Autodesk Fusion 360 part; units mm, degrees
(part 3 of 3)
  spline S31 degree 5 poles (22.8468, -21.88) (22.8333, -21.884) (22.8062, -21.8919) (22.7658, -21.904) (22.7119, -21.9202) (22.6448, -21.9407) (22.5778, -21.9615) (22.5111, -21.9825) (22.4444, -22.0039) (22.378, -22.0255) (22.3118, -22.0473) (22.2457, -22.0695) (22.1798, -22.0919) (22.1141, -22.1146) (22.0486, -22.1375) (21.9832, -22.1608) (21.9181, -22.1843) (21.8531, -22.2081) (21.7884, -22.2321) (21.7238, -22.2565) (21.6595, -22.2811) (21.5953, -22.306) (21.5314, -22.3312) (21.4676, -22.3567) (21.4041, -22.3825) (21.3408, -22.4086) (21.2777, -22.4349) (21.2148, -22.4616) (21.1522, -22.4885) (21.0897, -22.5157) (21.0275, -22.5433) (20.9655, -22.5711) (20.9038, -22.5992) (20.8423, -22.6276) (20.781, -22.6564) (20.72, -22.6854) (20.6592, -22.7148) (20.5987, -22.7444) (20.5384, -22.7744) (20.4784, -22.8047) (20.4187, -22.8353) (20.3592, -22.8662) (20.3, -22.8975) (20.2411, -22.9291) (20.1825, -22.9611) (20.1241, -22.9933) (20.066, -23.0259) (20.0083, -23.0589) (19.9508, -23.0921) (19.8936, -23.1258) (19.8368, -23.1598) (19.7803, -23.1942) (19.7242, -23.2289) (19.6685, -23.2641) (19.6131, -23.2997) (19.558, -23.3357) (19.5033, -23.372) (19.4489, -23.4086) (19.3948, -23.4456) (19.3412, -23.4831) (19.288, -23.521) (19.2355, -23.5596) (19.1835, -23.5987) (19.1321, -23.6385) (19.0813, -23.6788) (19.0309, -23.7195) (18.9808, -23.7605) (18.931, -23.8018) (18.8816, -23.8435) (18.8331, -23.886) (18.7858, -23.9297) (18.7495, -23.9661) (18.7233, -23.9943) (18.7062, -24.0136) (18.6978, -24.0233) knots -1 -1 -1 -1 -1 -1 -0.98571429 -0.97142857 -0.95714286 -0.94285714 -0.92857143 -0.91428571 -0.9 -0.88571429 -0.87142857 -0.85714286 -0.84285714 -0.82857143 -0.81428571 -0.8 -0.78571429 -0.77142857 -0.75714286 -0.74285714 -0.72857143 -0.71428571 -0.7 -0.68571429 -0.67142857 -0.65714286 -0.64285714 -0.62857143 -0.61428571 -0.6 -0.58571429 -0.57142857 -0.55714286 -0.54285714 -0.52857143 -0.51428571 -0.5 -0.48571429 -0.47142857 -0.45714286 -0.44285714 -0.42857143 -0.41428571 -0.4 -0.38571429 -0.37142857 -0.35714286 -0.34285714 -0.32857143 -0.31428571 -0.3 -0.28571429 -0.27142857 -0.25714286 -0.24285714 -0.22857143 -0.21428571 -0.2 -0.18571429 -0.17142857 -0.15714286 -0.14285714 -0.12857143 -0.11428571 -0.1 -0.08571429 -0.07142857 -0.05714286 -0.04285714 -0.02857143 -0.01428571 0 0 0 0 0 0
  line L31 (18.6978, -24.0233) -> (18.685, -24.0381)
  arc A63 (16.9379, -24.2063) -> (18.685, -24.0381) centre (17.7235, -23.2085) ccw
  arc A64 (16.9379, -24.2063) -> (16.3968, -23.7911) centre (0, -45.72) ccw
  arc A65 (16.1071, -22.0599) -> (16.3968, -23.7911) centre (17.1573, -22.774) ccw
  line L32 (16.1071, -22.0599) -> (16.1181, -22.0438)
  spline S32 degree 5 poles (16.1181, -22.0438) (16.1253, -22.0332) (16.1395, -22.0117) (16.16, -21.979) (16.1857, -21.9345) (16.2157, -21.8776) (16.2441, -21.8197) (16.2717, -21.7613) (16.2986, -21.7025) (16.3253, -21.6434) (16.3515, -21.5842) (16.3773, -21.5247) (16.4024, -21.4648) (16.4268, -21.4044) (16.4504, -21.3437) (16.4733, -21.2825) (16.4956, -21.221) (16.5174, -21.1592) (16.5387, -21.0972) (16.5596, -21.0349) (16.5801, -20.9724) (16.6001, -20.9097) (16.6197, -20.8468) (16.6388, -20.7836) (16.6574, -20.7201) (16.6755, -20.6564) (16.6932, -20.5925) (16.7105, -20.5284) (16.7273, -20.464) (16.7438, -20.3995) (16.7599, -20.3348) (16.7755, -20.2699) (16.7908, -20.2048) (16.8057, -20.1395) (16.8202, -20.0741) (16.8343, -20.0085) (16.848, -19.9426) (16.8614, -19.8767) (16.8743, -19.8105) (16.887, -19.7442) (16.8992, -19.6778) (16.9111, -19.6112) (16.9227, -19.5444) (16.9339, -19.4775) (16.9447, -19.4104) (16.9552, -19.3432) (16.9653, -19.2758) (16.9751, -19.2083) (16.9846, -19.1407) (16.9937, -19.0729) (17.0025, -19.005) (17.011, -18.937) (17.0191, -18.8688) (17.0269, -18.8005) (17.0343, -18.7321) (17.0415, -18.6636) (17.0483, -18.5949) (17.0548, -18.5262) (17.0609, -18.4573) (17.0668, -18.3883) (17.0723, -18.3191) (17.0776, -18.2499) (17.0825, -18.1806) (17.0871, -18.1111) (17.0913, -18.0416) (17.0953, -17.9719) (17.099, -17.9021) (17.1023, -17.8323) (17.1054, -17.7623) (17.1081, -17.6923) (17.1106, -17.6221) (17.1123, -17.5659) (17.1134, -17.5237) (17.1142, -17.4956) (17.1145, -17.4815) knots 0 0 0 0 0 0 0.01428571 0.02857143 0.04285714 0.05714286 0.07142857 0.08571429 0.1 0.11428571 0.12857143 0.14285714 0.15714286 0.17142857 0.18571429 0.2 0.21428571 0.22857143 0.24285714 0.25714286 0.27142857 0.28571429 0.3 0.31428571 0.32857143 0.34285714 0.35714286 0.37142857 0.38571429 0.4 0.41428571 0.42857143 0.44285714 0.45714286 0.47142857 0.48571429 0.5 0.51428571 0.52857143 0.54285714 0.55714286 0.57142857 0.58571429 0.6 0.61428571 0.62857143 0.64285714 0.65714286 0.67142857 0.68571429 0.7 0.71428571 0.72857143 0.74285714 0.75714286 0.77142857 0.78571429 0.8 0.81428571 0.82857143 0.84285714 0.85714286 0.87142857 0.88571429 0.9 0.91428571 0.92857143 0.94285714 0.95714286 0.97142857 0.98571429 1 1 1 1 1 1
  arc A66 (17.1145, -17.4815) -> (15.898, -16.7791) centre (0, -45.72) ccw
  spline S33 degree 5 poles (15.898, -16.7791) (15.886, -16.7865) (15.862, -16.8012) (15.826, -16.8233) (15.7782, -16.8528) (15.7187, -16.89) (15.6594, -16.9275) (15.6003, -16.9651) (15.5415, -17.0029) (15.4829, -17.041) (15.4246, -17.0792) (15.3665, -17.1177) (15.3086, -17.1564) (15.251, -17.1954) (15.1937, -17.2345) (15.1366, -17.2739) (15.0797, -17.3134) (15.0232, -17.3532) (14.9669, -17.3932) (14.9108, -17.4335) (14.855, -17.4739) (14.7995, -17.5146) (14.7443, -17.5555) (14.6893, -17.5966) (14.6346, -17.6379) (14.5802, -17.6795) (14.5261, -17.7213) (14.4722, -17.7633) (14.4187, -17.8055) (14.3654, -17.848) (14.3124, -17.8907) (14.2598, -17.9336) (14.2074, -17.9767) (14.1554, -18.0201) (14.1036, -18.0637) (14.0522, -18.1076) (14.0011, -18.1517) (13.9503, -18.196) (13.8998, -18.2405) (13.8497, -18.2853) (13.7999, -18.3303) (13.7505, -18.3756) (13.7014, -18.4211) (13.6527, -18.4669) (13.6043, -18.5129) (13.5563, -18.5592) (13.5087, -18.6057) (13.4614, -18.6525) (13.4145, -18.6995) (13.368, -18.7468) (13.3219, -18.7943) (13.2762, -18.8422) (13.231, -18.8903) (13.1863, -18.9387) (13.142, -18.9874) (13.0981, -19.0364) (13.0546, -19.0856) (13.0116, -19.1351) (12.969, -19.1849) (12.9268, -19.2349) (12.8853, -19.2853) (12.8445, -19.3362) (12.8044, -19.3874) (12.7651, -19.4392) (12.7264, -19.4912) (12.6883, -19.5436) (12.6505, -19.5962) (12.6131, -19.649) (12.5762, -19.702) (12.5403, -19.7556) (12.506, -19.8101) (12.4803, -19.8546) (12.4622, -19.8886) (12.4508, -19.9117) (12.4452, -19.9233) knots -1 -1 -1 -1 -1 -1 -0.98571429 -0.97142857 -0.95714286 -0.94285714 -0.92857143 -0.91428571 -0.9 -0.88571429 -0.87142857 -0.85714286 -0.84285714 -0.82857143 -0.81428571 -0.8 -0.78571429 -0.77142857 -0.75714286 -0.74285714 -0.72857143 -0.71428571 -0.7 -0.68571429 -0.67142857 -0.65714286 -0.64285714 -0.62857143 -0.61428571 -0.6 -0.58571429 -0.57142857 -0.55714286 -0.54285714 -0.52857143 -0.51428571 -0.5 -0.48571429 -0.47142857 -0.45714286 -0.44285714 -0.42857143 -0.41428571 -0.4 -0.38571429 -0.37142857 -0.35714286 -0.34285714 -0.32857143 -0.31428571 -0.3 -0.28571429 -0.27142857 -0.25714286 -0.24285714 -0.22857143 -0.21428571 -0.2 -0.18571429 -0.17142857 -0.15714286 -0.14285714 -0.12857143 -0.11428571 -0.1 -0.08571429 -0.07142857 -0.05714286 -0.04285714 -0.02857143 -0.01428571 0 0 0 0 0 0
  line L33 (12.4452, -19.9233) -> (12.4367, -19.9408)
  arc A67 (10.7926, -20.5555) -> (12.4367, -19.9408) centre (11.2931, -19.3883) ccw
  arc A68 (10.7926, -20.5555) -> (10.1625, -20.2945) centre (0, -45.72) ccw
  arc A69 (9.4346, -18.6973) -> (10.1625, -20.2945) centre (10.6338, -19.1152) ccw
  line L34 (9.4346, -18.6973) -> (9.441, -18.6789)
  spline S34 degree 5 poles (9.441, -18.6789) (9.4452, -18.6667) (9.4534, -18.6423) (9.4647, -18.6055) (9.478, -18.5558) (9.4923, -18.4931) (9.5048, -18.4298) (9.5162, -18.3662) (9.5271, -18.3024) (9.5375, -18.2385) (9.5476, -18.1745) (9.5571, -18.1103) (9.5658, -18.046) (9.5738, -17.9814) (9.5808, -17.9166) (9.5871, -17.8516) (9.5927, -17.7864) (9.5978, -17.7211) (9.6023, -17.6556) (9.6064, -17.5901) (9.61, -17.5244) (9.6131, -17.4587) (9.6157, -17.3928) (9.6178, -17.3268) (9.6193, -17.2607) (9.6204, -17.1945) (9.6209, -17.1282) (9.621, -17.0618) (9.6206, -16.9953) (9.6198, -16.9287) (9.6186, -16.862) (9.6169, -16.7953) (9.6149, -16.7284) (9.6123, -16.6615) (9.6094, -16.5946) (9.606, -16.5275) (9.6023, -16.4604) (9.5981, -16.3932) (9.5935, -16.326) (9.5885, -16.2587) (9.5832, -16.1913) (9.5774, -16.1239) (9.5713, -16.0564) (9.5648, -15.9889) (9.5579, -15.9213) (9.5506, -15.8536) (9.543, -15.7859) (9.535, -15.7182) (9.5266, -15.6504) (9.5179, -15.5826) (9.5088, -15.5147) (9.4994, -15.4468) (9.4896, -15.3789) (9.4794, -15.3109) (9.4689, -15.2429) (9.4581, -15.1749) (9.4469, -15.1068) (9.4354, -15.0387) (9.4235, -14.9705) (9.4113, -14.9024) (9.3987, -14.8342) (9.3859, -14.7659) (9.3727, -14.6977) (9.3591, -14.6294) (9.3453, -14.5611) (9.3311, -14.4928) (9.3166, -14.4245) (9.3017, -14.3561) (9.2866, -14.2878) (9.2711, -14.2194) (9.2553, -14.151) (9.2424, -14.0962) (9.2326, -14.0552) (9.226, -14.0278) (9.2227, -14.0141) knots 0 0 0 0 0 0 0.01428571 0.02857143 0.04285714 0.05714286 0.07142857 0.08571429 0.1 0.11428571 0.12857143 0.14285714 0.15714286 0.17142857 0.18571429 0.2 0.21428571 0.22857143 0.24285714 0.25714286 0.27142857 0.28571429 0.3 0.31428571 0.32857143 0.34285714 0.35714286 0.37142857 0.38571429 0.4 0.41428571 0.42857143 0.44285714 0.45714286 0.47142857 0.48571429 0.5 0.51428571 0.52857143 0.54285714 0.55714286 0.57142857 0.58571429 0.6 0.61428571 0.62857143 0.64285714 0.65714286 0.67142857 0.68571429 0.7 0.71428571 0.72857143 0.74285714 0.75714286 0.77142857 0.78571429 0.8 0.81428571 0.82857143 0.84285714 0.85714286 0.87142857 0.88571429 0.9 0.91428571 0.92857143 0.94285714 0.95714286 0.97142857 0.98571429 1 1 1 1 1 1
  arc A70 (9.2227, -14.0141) -> (7.8659, -13.6506) centre (0, -45.72) ccw
  spline S35 degree 5 poles (7.8659, -13.6506) (7.8562, -13.6608) (7.8368, -13.6812) (7.8077, -13.7118) (7.7692, -13.7528) (7.7213, -13.8041) (7.6737, -13.8556) (7.6264, -13.9072) (7.5794, -13.959) (7.5327, -14.0109) (7.4862, -14.063) (7.4401, -14.1152) (7.3942, -14.1676) (7.3486, -14.2201) (7.3034, -14.2727) (7.2584, -14.3255) (7.2138, -14.3784) (7.1694, -14.4315) (7.1254, -14.4847) (7.0816, -14.5381) (7.0382, -14.5916) (6.9951, -14.6453) (6.9523, -14.6991) (6.9099, -14.753) (6.8678, -14.8071) (6.826, -14.8613) (6.7845, -14.9157) (6.7433, -14.9702) (6.7026, -15.0248) (6.6621, -15.0796) (6.622, -15.1346) (6.5822, -15.1897) (6.5428, -15.2449) (6.5038, -15.3003) (6.4651, -15.3558) (6.4268, -15.4115) (6.3888, -15.4673) (6.3512, -15.5232) (6.314, -15.5793) (6.2772, -15.6356) (6.2407, -15.6919) (6.2047, -15.7485) (6.1691, -15.8051) (6.1338, -15.862) (6.099, -15.9189) (6.0646, -15.9761) (6.0307, -16.0333) (5.9971, -16.0907) (5.964, -16.1483) (5.9313, -16.206) (5.8991, -16.2639) (5.8673, -16.3219) (5.8361, -16.3801) (5.8054, -16.4384) (5.7753, -16.4969) (5.7456, -16.5556) (5.7163, -16.6144) (5.6875, -16.6733) (5.6592, -16.7324) (5.6315, -16.7917) (5.6045, -16.8511) (5.5782, -16.9108) (5.5528, -16.9707) (5.5282, -17.0308) (5.5043, -17.0911) (5.481, -17.1516) (5.4581, -17.2122) (5.4356, -17.2728) (5.4137, -17.3336) (5.3929, -17.3947) (5.3739, -17.4561) (5.3606, -17.5058) (5.352, -17.5434) (5.3468, -17.5686) (5.3444, -17.5812) knots -1 -1 -1 -1 -1 -1 -0.98571429 -0.97142857 -0.95714286 -0.94285714 -0.92857143 -0.91428571 -0.9 -0.88571429 -0.87142857 -0.85714286 -0.84285714 -0.82857143 -0.81428571 -0.8 -0.78571429 -0.77142857 -0.75714286 -0.74285714 -0.72857143 -0.71428571 -0.7 -0.68571429 -0.67142857 -0.65714286 -0.64285714 -0.62857143 -0.61428571 -0.6 -0.58571429 -0.57142857 -0.55714286 -0.54285714 -0.52857143 -0.51428571 -0.5 -0.48571429 -0.47142857 -0.45714286 -0.44285714 -0.42857143 -0.41428571 -0.4 -0.38571429 -0.37142857 -0.35714286 -0.34285714 -0.32857143 -0.31428571 -0.3 -0.28571429 -0.27142857 -0.25714286 -0.24285714 -0.22857143 -0.21428571 -0.2 -0.18571429 -0.17142857 -0.15714286 -0.14285714 -0.12857143 -0.11428571 -0.1 -0.08571429 -0.07142857 -0.05714286 -0.04285714 -0.02857143 -0.01428571 0 0 0 0 0 0
  line L35 (5.3444, -17.5812) -> (5.3408, -17.6004)
  arc A71 (3.9118, -18.6197) -> (5.3408, -17.6004) centre (4.0932, -17.3627) ccw
  arc A72 (3.9118, -18.6197) -> (3.2356, -18.5306) centre (0, -45.72) ccw
  arc A73 (2.1191, -17.1763) -> (3.2356, -18.5306) centre (3.3857, -17.2695) ccw
  line L36 (2.1191, -17.1763) -> (2.1205, -17.1568)
  spline S36 degree 5 poles (2.1205, -17.1568) (2.1215, -17.1439) (2.1231, -17.1183) (2.1244, -17.0797) (2.1245, -17.0283) (2.122, -16.964) (2.1177, -16.8997) (2.1123, -16.8353) (2.1063, -16.7709) (2.0998, -16.7065) (2.093, -16.642) (2.0855, -16.5776) (2.0773, -16.5131) (2.0683, -16.4487) (2.0583, -16.3843) (2.0476, -16.3198) (2.0361, -16.2554) (2.0241, -16.191) (2.0115, -16.1266) (1.9985, -16.0623) (1.985, -15.9979) (1.971, -15.9336) (1.9565, -15.8693) (1.9414, -15.805) (1.9257, -15.7408) (1.9096, -15.6765) (1.893, -15.6123) (1.8759, -15.5482) (1.8583, -15.484) (1.8403, -15.4199) (1.8219, -15.3558) (1.803, -15.2918) (1.7837, -15.2278) (1.7639, -15.1638) (1.7437, -15.0999) (1.7231, -15.036) (1.7021, -14.9722) (1.6807, -14.9083) (1.6589, -14.8446) (1.6367, -14.7808) (1.614, -14.7172) (1.591, -14.6535) (1.5677, -14.5899) (1.5439, -14.5264) (1.5197, -14.4629) (1.4952, -14.3994) (1.4703, -14.336) (1.4451, -14.2727) (1.4194, -14.2094) (1.3935, -14.1461) (1.3671, -14.0829) (1.3404, -14.0198) (1.3134, -13.9567) (1.286, -13.8936) (1.2582, -13.8307) (1.2301, -13.7677) (1.2017, -13.7049) (1.1729, -13.6421) (1.1438, -13.5793) (1.1144, -13.5166) (1.0846, -13.454) (1.0546, -13.3914) (1.0241, -13.3289) (0.9934, -13.2665) (0.9623, -13.2041) (0.9309, -13.1418) (0.8992, -13.0795) (0.8672, -13.0174) (0.8349, -12.9552) (0.8022, -12.8932) (0.7693, -12.8312) (0.7426, -12.7817) (0.7225, -12.7446) (0.7091, -12.7198) (0.7023, -12.7075) knots 0 0 0 0 0 0 0.01428571 0.02857143 0.04285714 0.05714286 0.07142857 0.08571429 0.1 0.11428571 0.12857143 0.14285714 0.15714286 0.17142857 0.18571429 0.2 0.21428571 0.22857143 0.24285714 0.25714286 0.27142857 0.28571429 0.3 0.31428571 0.32857143 0.34285714 0.35714286 0.37142857 0.38571429 0.4 0.41428571 0.42857143 0.44285714 0.45714286 0.47142857 0.48571429 0.5 0.51428571 0.52857143 0.54285714 0.55714286 0.57142857 0.58571429 0.6 0.61428571 0.62857143 0.64285714 0.65714286 0.67142857 0.68571429 0.7 0.71428571 0.72857143 0.74285714 0.75714286 0.77142857 0.78571429 0.8 0.81428571 0.82857143 0.84285714 0.85714286 0.87142857 0.88571429 0.9 0.91428571 0.92857143 0.94285714 0.95714286 0.97142857 0.98571429 1 1 1 1 1 1
  arc A74 (0.7023, -12.7075) -> (-0.7023, -12.7075) centre (0, -45.72) ccw
  spline S37 degree 5 poles (-0.7023, -12.7075) (-0.7091, -12.7198) (-0.7225, -12.7446) (-0.7426, -12.7817) (-0.7693, -12.8312) (-0.8022, -12.8932) (-0.8349, -12.9552) (-0.8672, -13.0174) (-0.8992, -13.0795) (-0.9309, -13.1418) (-0.9623, -13.2041) (-0.9934, -13.2665) (-1.0241, -13.3289) (-1.0546, -13.3914) (-1.0846, -13.454) (-1.1144, -13.5166) (-1.1438, -13.5793) (-1.1729, -13.6421) (-1.2017, -13.7049) (-1.2301, -13.7677) (-1.2582, -13.8307) (-1.286, -13.8936) (-1.3134, -13.9567) (-1.3404, -14.0198) (-1.3671, -14.0829) (-1.3935, -14.1461) (-1.4194, -14.2094) (-1.4451, -14.2727) (-1.4703, -14.336) (-1.4952, -14.3994) (-1.5197, -14.4629) (-1.5439, -14.5264) (-1.5677, -14.5899) (-1.591, -14.6535) (-1.614, -14.7172) (-1.6367, -14.7808) (-1.6589, -14.8446) (-1.6807, -14.9083) (-1.7021, -14.9722) (-1.7231, -15.036) (-1.7437, -15.0999) (-1.7639, -15.1638) (-1.7837, -15.2278) (-1.803, -15.2918) (-1.8219, -15.3558) (-1.8403, -15.4199) (-1.8583, -15.484) (-1.8759, -15.5482) (-1.893, -15.6123) (-1.9096, -15.6765) (-1.9257, -15.7408) (-1.9414, -15.805) (-1.9565, -15.8693) (-1.971, -15.9336) (-1.985, -15.9979) (-1.9985, -16.0623) (-2.0115, -16.1266) (-2.0241, -16.191) (-2.0361, -16.2554) (-2.0476, -16.3198) (-2.0583, -16.3843) (-2.0683, -16.4487) (-2.0773, -16.5131) (-2.0855, -16.5776) (-2.093, -16.642) (-2.0998, -16.7065) (-2.1063, -16.7709) (-2.1123, -16.8353) (-2.1177, -16.8997) (-2.122, -16.964) (-2.1245, -17.0283) (-2.1244, -17.0797) (-2.1231, -17.1183) (-2.1215, -17.1439) (-2.1205, -17.1568) knots -1 -1 -1 -1 -1 -1 -0.98571429 -0.97142857 -0.95714286 -0.94285714 -0.92857143 -0.91428571 -0.9 -0.88571429 -0.87142857 -0.85714286 -0.84285714 -0.82857143 -0.81428571 -0.8 -0.78571429 -0.77142857 -0.75714286 -0.74285714 -0.72857143 -0.71428571 -0.7 -0.68571429 -0.67142857 -0.65714286 -0.64285714 -0.62857143 -0.61428571 -0.6 -0.58571429 -0.57142857 -0.55714286 -0.54285714 -0.52857143 -0.51428571 -0.5 -0.48571429 -0.47142857 -0.45714286 -0.44285714 -0.42857143 -0.41428571 -0.4 -0.38571429 -0.37142857 -0.35714286 -0.34285714 -0.32857143 -0.31428571 -0.3 -0.28571429 -0.27142857 -0.25714286 -0.24285714 -0.22857143 -0.21428571 -0.2 -0.18571429 -0.17142857 -0.15714286 -0.14285714 -0.12857143 -0.11428571 -0.1 -0.08571429 -0.07142857 -0.05714286 -0.04285714 -0.02857143 -0.01428571 0 0 0 0 0 0
  line L37 (-2.1205, -17.1568) -> (-2.1191, -17.1763)
  arc A75 (-3.2356, -18.5306) -> (-2.1191, -17.1763) centre (-3.3857, -17.2695) ccw
  arc A76 (-3.2356, -18.5306) -> (-3.9118, -18.6197) centre (0, -45.72) ccw
  arc A77 (-5.3408, -17.6004) -> (-3.9118, -18.6197) centre (-4.0932, -17.3627) ccw
  line L38 (-5.3408, -17.6004) -> (-5.3444, -17.5812)
  spline S38 degree 5 poles (-5.3444, -17.5812) (-5.3468, -17.5686) (-5.352, -17.5434) (-5.3606, -17.5058) (-5.3739, -17.4561) (-5.3929, -17.3947) (-5.4137, -17.3336) (-5.4356, -17.2728) (-5.4581, -17.2122) (-5.481, -17.1516) (-5.5043, -17.0911) (-5.5282, -17.0308) (-5.5528, -16.9707) (-5.5782, -16.9108) (-5.6045, -16.8511) (-5.6315, -16.7917) (-5.6592, -16.7324) (-5.6875, -16.6733) (-5.7163, -16.6144) (-5.7456, -16.5556) (-5.7753, -16.4969) (-5.8054, -16.4384) (-5.8361, -16.3801) (-5.8673, -16.3219) (-5.8991, -16.2639) (-5.9313, -16.206) (-5.964, -16.1483) (-5.9971, -16.0907) (-6.0307, -16.0333) (-6.0646, -15.9761) (-6.099, -15.9189) (-6.1338, -15.862) (-6.1691, -15.8051) (-6.2047, -15.7485) (-6.2407, -15.6919) (-6.2772, -15.6356) (-6.314, -15.5793) (-6.3512, -15.5232) (-6.3888, -15.4673) (-6.4268, -15.4115) (-6.4651, -15.3558) (-6.5038, -15.3003) (-6.5428, -15.2449) (-6.5822, -15.1897) (-6.622, -15.1346) (-6.6621, -15.0796) (-6.7026, -15.0248) (-6.7433, -14.9702) (-6.7845, -14.9157) (-6.826, -14.8613) (-6.8678, -14.8071) (-6.9099, -14.753) (-6.9523, -14.6991) (-6.9951, -14.6453) (-7.0382, -14.5916) (-7.0816, -14.5381) (-7.1254, -14.4847) (-7.1694, -14.4315) (-7.2138, -14.3784) (-7.2584, -14.3255) (-7.3034, -14.2727) (-7.3486, -14.2201) (-7.3942, -14.1676) (-7.4401, -14.1152) (-7.4862, -14.063) (-7.5327, -14.0109) (-7.5794, -13.959) (-7.6264, -13.9072) (-7.6737, -13.8556) (-7.7213, -13.8041) (-7.7692, -13.7528) (-7.8077, -13.7118) (-7.8368, -13.6812) (-7.8562, -13.6608) (-7.8659, -13.6506) knots 0 0 0 0 0 0 0.01428571 0.02857143 0.04285714 0.05714286 0.07142857 0.08571429 0.1 0.11428571 0.12857143 0.14285714 0.15714286 0.17142857 0.18571429 0.2 0.21428571 0.22857143 0.24285714 0.25714286 0.27142857 0.28571429 0.3 0.31428571 0.32857143 0.34285714 0.35714286 0.37142857 0.38571429 0.4 0.41428571 0.42857143 0.44285714 0.45714286 0.47142857 0.48571429 0.5 0.51428571 0.52857143 0.54285714 0.55714286 0.57142857 0.58571429 0.6 0.61428571 0.62857143 0.64285714 0.65714286 0.67142857 0.68571429 0.7 0.71428571 0.72857143 0.74285714 0.75714286 0.77142857 0.78571429 0.8 0.81428571 0.82857143 0.84285714 0.85714286 0.87142857 0.88571429 0.9 0.91428571 0.92857143 0.94285714 0.95714286 0.97142857 0.98571429 1 1 1 1 1 1
  arc A78 (-7.8659, -13.6506) -> (-9.2227, -14.0141) centre (0, -45.72) ccw
  spline S39 degree 5 poles (-9.2227, -14.0141) (-9.226, -14.0278) (-9.2326, -14.0552) (-9.2424, -14.0962) (-9.2553, -14.151) (-9.2711, -14.2194) (-9.2866, -14.2878) (-9.3017, -14.3561) (-9.3166, -14.4245) (-9.3311, -14.4928) (-9.3453, -14.5611) (-9.3591, -14.6294) (-9.3727, -14.6977) (-9.3859, -14.7659) (-9.3987, -14.8342) (-9.4113, -14.9024) (-9.4235, -14.9705) (-9.4354, -15.0387) (-9.4469, -15.1068) (-9.4581, -15.1749) (-9.4689, -15.2429) (-9.4794, -15.3109) (-9.4896, -15.3789) (-9.4994, -15.4468) (-9.5088, -15.5147) (-9.5179, -15.5826) (-9.5266, -15.6504) (-9.535, -15.7182) (-9.543, -15.7859) (-9.5506, -15.8536) (-9.5579, -15.9213) (-9.5648, -15.9889) (-9.5713, -16.0564) (-9.5774, -16.1239) (-9.5832, -16.1913) (-9.5885, -16.2587) (-9.5935, -16.326) (-9.5981, -16.3932) (-9.6023, -16.4604) (-9.606, -16.5275) (-9.6094, -16.5946) (-9.6123, -16.6615) (-9.6149, -16.7284) (-9.6169, -16.7953) (-9.6186, -16.862) (-9.6198, -16.9287) (-9.6206, -16.9953) (-9.621, -17.0618) (-9.6209, -17.1282) (-9.6204, -17.1945) (-9.6193, -17.2607) (-9.6178, -17.3268) (-9.6157, -17.3928) (-9.6131, -17.4587) (-9.61, -17.5244) (-9.6064, -17.5901) (-9.6023, -17.6556) (-9.5978, -17.7211) (-9.5927, -17.7864) (-9.5871, -17.8516) (-9.5808, -17.9166) (-9.5738, -17.9814) (-9.5658, -18.046) (-9.5571, -18.1103) (-9.5476, -18.1745) (-9.5375, -18.2385) (-9.5271, -18.3024) (-9.5162, -18.3662) (-9.5048, -18.4298) (-9.4923, -18.4931) (-9.478, -18.5558) (-9.4647, -18.6055) (-9.4534, -18.6423) (-9.4452, -18.6667) (-9.441, -18.6789) knots -1 -1 -1 -1 -1 -1 -0.98571429 -0.97142857 -0.95714286 -0.94285714 -0.92857143 -0.91428571 -0.9 -0.88571429 -0.87142857 -0.85714286 -0.84285714 -0.82857143 -0.81428571 -0.8 -0.78571429 -0.77142857 -0.75714286 -0.74285714 -0.72857143 -0.71428571 -0.7 -0.68571429 -0.67142857 -0.65714286 -0.64285714 -0.62857143 -0.61428571 -0.6 -0.58571429 -0.57142857 -0.55714286 -0.54285714 -0.52857143 -0.51428571 -0.5 -0.48571429 -0.47142857 -0.45714286 -0.44285714 -0.42857143 -0.41428571 -0.4 -0.38571429 -0.37142857 -0.35714286 -0.34285714 -0.32857143 -0.31428571 -0.3 -0.28571429 -0.27142857 -0.25714286 -0.24285714 -0.22857143 -0.21428571 -0.2 -0.18571429 -0.17142857 -0.15714286 -0.14285714 -0.12857143 -0.11428571 -0.1 -0.08571429 -0.07142857 -0.05714286 -0.04285714 -0.02857143 -0.01428571 0 0 0 0 0 0
  line L39 (-9.441, -18.6789) -> (-9.4346, -18.6973)
  arc A79 (-10.1625, -20.2945) -> (-9.4346, -18.6973) centre (-10.6338, -19.1152) ccw
  arc A80 (-10.1625, -20.2945) -> (-10.7926, -20.5555) centre (0, -45.72) ccw
  arc A81 (-12.4367, -19.9408) -> (-10.7926, -20.5555) centre (-11.2931, -19.3883) ccw
  line L40 (-12.4367, -19.9408) -> (-12.4452, -19.9233)
  spline S40 degree 5 poles (-12.4452, -19.9233) (-12.4508, -19.9117) (-12.4622, -19.8886) (-12.4803, -19.8546) (-12.506, -19.8101) (-12.5403, -19.7556) (-12.5762, -19.702) (-12.6131, -19.649) (-12.6505, -19.5962) (-12.6883, -19.5436) (-12.7264, -19.4912) (-12.7651, -19.4392) (-12.8044, -19.3874) (-12.8445, -19.3362) (-12.8853, -19.2853) (-12.9268, -19.2349) (-12.969, -19.1849) (-13.0116, -19.1351) (-13.0546, -19.0856) (-13.0981, -19.0364) (-13.142, -18.9874) (-13.1863, -18.9387) (-13.231, -18.8903) (-13.2762, -18.8422) (-13.3219, -18.7943) (-13.368, -18.7468) (-13.4145, -18.6995) (-13.4614, -18.6525) (-13.5087, -18.6057) (-13.5563, -18.5592) (-13.6043, -18.5129) (-13.6527, -18.4669) (-13.7014, -18.4211) (-13.7505, -18.3756) (-13.7999, -18.3303) (-13.8497, -18.2853) (-13.8998, -18.2405) (-13.9503, -18.196) (-14.0011, -18.1517) (-14.0522, -18.1076) (-14.1036, -18.0637) (-14.1554, -18.0201) (-14.2074, -17.9767) (-14.2598, -17.9336) (-14.3124, -17.8907) (-14.3654, -17.848) (-14.4187, -17.8055) (-14.4722, -17.7633) (-14.5261, -17.7213) (-14.5802, -17.6795) (-14.6346, -17.6379) (-14.6893, -17.5966) (-14.7443, -17.5555) (-14.7995, -17.5146) (-14.855, -17.4739) (-14.9108, -17.4335) (-14.9669, -17.3932) (-15.0232, -17.3532) (-15.0797, -17.3134) (-15.1366, -17.2739) (-15.1937, -17.2345) (-15.251, -17.1954) (-15.3086, -17.1564) (-15.3665, -17.1177) (-15.4246, -17.0792) (-15.4829, -17.041) (-15.5415, -17.0029) (-15.6003, -16.9651) (-15.6594, -16.9275) (-15.7187, -16.89) (-15.7782, -16.8528) (-15.826, -16.8233) (-15.862, -16.8012) (-15.886, -16.7865) (-15.898, -16.7791) knots 0 0 0 0 0 0 0.01428571 0.02857143 0.04285714 0.05714286 0.07142857 0.08571429 0.1 0.11428571 0.12857143 0.14285714 0.15714286 0.17142857 0.18571429 0.2 0.21428571 0.22857143 0.24285714 0.25714286 0.27142857 0.28571429 0.3 0.31428571 0.32857143 0.34285714 0.35714286 0.37142857 0.38571429 0.4 0.41428571 0.42857143 0.44285714 0.45714286 0.47142857 0.48571429 0.5 0.51428571 0.52857143 0.54285714 0.55714286 0.57142857 0.58571429 0.6 0.61428571 0.62857143 0.64285714 0.65714286 0.67142857 0.68571429 0.7 0.71428571 0.72857143 0.74285714 0.75714286 0.77142857 0.78571429 0.8 0.81428571 0.82857143 0.84285714 0.85714286 0.87142857 0.88571429 0.9 0.91428571 0.92857143 0.94285714 0.95714286 0.97142857 0.98571429 1 1 1 1 1 1
  arc A82 (-15.898, -16.7791) -> (-17.1145, -17.4815) centre (0, -45.72) ccw
  spline S41 degree 5 poles (-17.1145, -17.4815) (-17.1142, -17.4956) (-17.1134, -17.5237) (-17.1123, -17.5659) (-17.1106, -17.6221) (-17.1081, -17.6923) (-17.1054, -17.7623) (-17.1023, -17.8323) (-17.099, -17.9021) (-17.0953, -17.9719) (-17.0913, -18.0416) (-17.0871, -18.1111) (-17.0825, -18.1806) (-17.0776, -18.2499) (-17.0723, -18.3191) (-17.0668, -18.3883) (-17.0609, -18.4573) (-17.0548, -18.5262) (-17.0483, -18.5949) (-17.0415, -18.6636) (-17.0343, -18.7321) (-17.0269, -18.8005) (-17.0191, -18.8688) (-17.011, -18.937) (-17.0025, -19.005) (-16.9937, -19.0729) (-16.9846, -19.1407) (-16.9751, -19.2083) (-16.9653, -19.2758) (-16.9552, -19.3432) (-16.9447, -19.4104) (-16.9339, -19.4775) (-16.9227, -19.5444) (-16.9111, -19.6112) (-16.8992, -19.6778) (-16.887, -19.7442) (-16.8743, -19.8105) (-16.8614, -19.8767) (-16.848, -19.9426) (-16.8343, -20.0085) (-16.8202, -20.0741) (-16.8057, -20.1395) (-16.7908, -20.2048) (-16.7755, -20.2699) (-16.7599, -20.3348) (-16.7438, -20.3995) (-16.7273, -20.464) (-16.7105, -20.5284) (-16.6932, -20.5925) (-16.6755, -20.6564) (-16.6574, -20.7201) (-16.6388, -20.7836) (-16.6197, -20.8468) (-16.6001, -20.9097) (-16.5801, -20.9724) (-16.5596, -21.0349) (-16.5387, -21.0972) (-16.5174, -21.1592) (-16.4956, -21.221) (-16.4733, -21.2825) (-16.4504, -21.3437) (-16.4268, -21.4044) (-16.4024, -21.4648) (-16.3773, -21.5247) (-16.3515, -21.5842) (-16.3253, -21.6434) (-16.2986, -21.7025) (-16.2717, -21.7613) (-16.2441, -21.8197) (-16.2157, -21.8776) (-16.1857, -21.9345) (-16.16, -21.979) (-16.1395, -22.0117) (-16.1253, -22.0332) (-16.1181, -22.0438) knots -1 -1 -1 -1 -1 -1 -0.98571429 -0.97142857 -0.95714286 -0.94285714 -0.92857143 -0.91428571 -0.9 -0.88571429 -0.87142857 -0.85714286 -0.84285714 -0.82857143 -0.81428571 -0.8 -0.78571429 -0.77142857 -0.75714286 -0.74285714 -0.72857143 -0.71428571 -0.7 -0.68571429 -0.67142857 -0.65714286 -0.64285714 -0.62857143 -0.61428571 -0.6 -0.58571429 -0.57142857 -0.55714286 -0.54285714 -0.52857143 -0.51428571 -0.5 -0.48571429 -0.47142857 -0.45714286 -0.44285714 -0.42857143 -0.41428571 -0.4 -0.38571429 -0.37142857 -0.35714286 -0.34285714 -0.32857143 -0.31428571 -0.3 -0.28571429 -0.27142857 -0.25714286 -0.24285714 -0.22857143 -0.21428571 -0.2 -0.18571429 -0.17142857 -0.15714286 -0.14285714 -0.12857143 -0.11428571 -0.1 -0.08571429 -0.07142857 -0.05714286 -0.04285714 -0.02857143 -0.01428571 0 0 0 0 0 0
  line L41 (-16.1181, -22.0438) -> (-16.1071, -22.0599)
  arc A83 (-16.3968, -23.7911) -> (-16.1071, -22.0599) centre (-17.1573, -22.774) ccw
  arc A84 (-16.3968, -23.7911) -> (-16.9379, -24.2063) centre (0, -45.72) ccw
  arc A85 (-18.685, -24.0381) -> (-16.9379, -24.2063) centre (-17.7235, -23.2085) ccw
  line L42 (-18.685, -24.0381) -> (-18.6978, -24.0233)
  spline S42 degree 5 poles (-18.6978, -24.0233) (-18.7062, -24.0136) (-18.7233, -23.9943) (-18.7495, -23.9661) (-18.7858, -23.9297) (-18.8331, -23.886) (-18.8816, -23.8435) (-18.931, -23.8018) (-18.9808, -23.7605) (-19.0309, -23.7195) (-19.0813, -23.6788) (-19.1321, -23.6385) (-19.1835, -23.5987) (-19.2355, -23.5596) (-19.288, -23.521) (-19.3412, -23.4831) (-19.3948, -23.4456) (-19.4489, -23.4086) (-19.5033, -23.372) (-19.558, -23.3357) (-19.6131, -23.2997) (-19.6685, -23.2641) (-19.7242, -23.2289) (-19.7803, -23.1942) (-19.8368, -23.1598) (-19.8936, -23.1258) (-19.9508, -23.0921) (-20.0083, -23.0589) (-20.066, -23.0259) (-20.1241, -22.9933) (-20.1825, -22.9611) (-20.2411, -22.9291) (-20.3, -22.8975) (-20.3592, -22.8662) (-20.4187, -22.8353) (-20.4784, -22.8047) (-20.5384, -22.7744) (-20.5987, -22.7444) (-20.6592, -22.7148) (-20.72, -22.6854) (-20.781, -22.6564) (-20.8423, -22.6276) (-20.9038, -22.5992) (-20.9655, -22.5711) (-21.0275, -22.5433) (-21.0897, -22.5157) (-21.1522, -22.4885) (-21.2148, -22.4616) (-21.2777, -22.4349) (-21.3408, -22.4086) (-21.4041, -22.3825) (-21.4676, -22.3567) (-21.5314, -22.3312) (-21.5953, -22.306) (-21.6595, -22.2811) (-21.7238, -22.2565) (-21.7884, -22.2321) (-21.8531, -22.2081) (-21.9181, -22.1843) (-21.9832, -22.1608) (-22.0486, -22.1375) (-22.1141, -22.1146) (-22.1798, -22.0919) (-22.2457, -22.0695) (-22.3118, -22.0473) (-22.378, -22.0255) (-22.4444, -22.0039) (-22.5111, -21.9825) (-22.5778, -21.9615) (-22.6448, -21.9407) (-22.7119, -21.9202) (-22.7658, -21.904) (-22.8062, -21.8919) (-22.8333, -21.884) (-22.8468, -21.88) knots 0 0 0 0 0 0 0.01428571 0.02857143 0.04285714 0.05714286 0.07142857 0.08571429 0.1 0.11428571 0.12857143 0.14285714 0.15714286 0.17142857 0.18571429 0.2 0.21428571 0.22857143 0.24285714 0.25714286 0.27142857 0.28571429 0.3 0.31428571 0.32857143 0.34285714 0.35714286 0.37142857 0.38571429 0.4 0.41428571 0.42857143 0.44285714 0.45714286 0.47142857 0.48571429 0.5 0.51428571 0.52857143 0.54285714 0.55714286 0.57142857 0.58571429 0.6 0.61428571 0.62857143 0.64285714 0.65714286 0.67142857 0.68571429 0.7 0.71428571 0.72857143 0.74285714 0.75714286 0.77142857 0.78571429 0.8 0.81428571 0.82857143 0.84285714 0.85714286 0.87142857 0.88571429 0.9 0.91428571 0.92857143 0.94285714 0.95714286 0.97142857 0.98571429 1 1 1 1 1 1
  arc A86 (-22.8468, -21.88) -> (-23.84, -22.8732) centre (0, -45.72) ccw
  spline S43 degree 5 poles (-23.84, -22.8732) (-23.836, -22.8867) (-23.8281, -22.9138) (-23.816, -22.9542) (-23.7998, -23.0081) (-23.7793, -23.0752) (-23.7585, -23.1422) (-23.7375, -23.2089) (-23.7161, -23.2756) (-23.6945, -23.342) (-23.6727, -23.4082) (-23.6505, -23.4743) (-23.6281, -23.5402) (-23.6054, -23.6059) (-23.5825, -23.6714) (-23.5592, -23.7368) (-23.5357, -23.8019) (-23.5119, -23.8669) (-23.4879, -23.9316) (-23.4635, -23.9962) (-23.4389, -24.0605) (-23.414, -24.1247) (-23.3888, -24.1886) (-23.3633, -24.2524) (-23.3375, -24.3159) (-23.3114, -24.3792) (-23.2851, -24.4423) (-23.2584, -24.5052) (-23.2315, -24.5678) (-23.2043, -24.6303) (-23.1767, -24.6925) (-23.1489, -24.7545) (-23.1208, -24.8162) (-23.0924, -24.8777) (-23.0636, -24.939) (-23.0346, -25) (-23.0052, -25.0608) (-22.9756, -25.1213) (-22.9456, -25.1816) (-22.9153, -25.2416) (-22.8847, -25.3013) (-22.8538, -25.3608) (-22.8225, -25.42) (-22.7909, -25.4789) (-22.7589, -25.5375) (-22.7267, -25.5959) (-22.6941, -25.654) (-22.6611, -25.7117) (-22.6279, -25.7692) (-22.5942, -25.8264) (-22.5602, -25.8832) (-22.5258, -25.9397) (-22.4911, -25.9958) (-22.4559, -26.0515) (-22.4203, -26.1069) (-22.3843, -26.162) (-22.348, -26.2167) (-22.3114, -26.2711) (-22.2744, -26.3252) (-22.2369, -26.3788) (-22.199, -26.432) (-22.1604, -26.4845) (-22.1213, -26.5365) (-22.0815, -26.5879) (-22.0412, -26.6387) (-22.0005, -26.6891) (-21.9595, -26.7392) (-21.9182, -26.789) (-21.8765, -26.8384) (-21.834, -26.8869) (-21.7903, -26.9342) (-21.7539, -26.9705) (-21.7257, -26.9967) (-21.7064, -27.0138) (-21.6967, -27.0222) knots -1 -1 -1 -1 -1 -1 -0.98571429 -0.97142857 -0.95714286 -0.94285714 -0.92857143 -0.91428571 -0.9 -0.88571429 -0.87142857 -0.85714286 -0.84285714 -0.82857143 -0.81428571 -0.8 -0.78571429 -0.77142857 -0.75714286 -0.74285714 -0.72857143 -0.71428571 -0.7 -0.68571429 -0.67142857 -0.65714286 -0.64285714 -0.62857143 -0.61428571 -0.6 -0.58571429 -0.57142857 -0.55714286 -0.54285714 -0.52857143 -0.51428571 -0.5 -0.48571429 -0.47142857 -0.45714286 -0.44285714 -0.42857143 -0.41428571 -0.4 -0.38571429 -0.37142857 -0.35714286 -0.34285714 -0.32857143 -0.31428571 -0.3 -0.28571429 -0.27142857 -0.25714286 -0.24285714 -0.22857143 -0.21428571 -0.2 -0.18571429 -0.17142857 -0.15714286 -0.14285714 -0.12857143 -0.11428571 -0.1 -0.08571429 -0.07142857 -0.05714286 -0.04285714 -0.02857143 -0.01428571 0 0 0 0 0 0
  line L43 (-21.6967, -27.0222) -> (-21.6819, -27.035)
  arc A87 (-21.5137, -28.7821) -> (-21.6819, -27.035) centre (-22.5115, -27.9965) ccw
  arc A88 (-21.5137, -28.7821) -> (-21.9289, -29.3232) centre (0, -45.72) ccw
  arc A89 (-23.6601, -29.6129) -> (-21.9289, -29.3232) centre (-22.946, -28.5627) ccw
  line L44 (-23.6601, -29.6129) -> (-23.6762, -29.6019)
  spline S44 degree 5 poles (-23.6762, -29.6019) (-23.6868, -29.5947) (-23.7083, -29.5805) (-23.741, -29.56) (-23.7855, -29.5343) (-23.8424, -29.5043) (-23.9003, -29.4759) (-23.9587, -29.4483) (-24.0175, -29.4214) (-24.0766, -29.3947) (-24.1358, -29.3685) (-24.1953, -29.3427) (-24.2552, -29.3176) (-24.3156, -29.2932) (-24.3763, -29.2696) (-24.4375, -29.2467) (-24.499, -29.2244) (-24.5608, -29.2026) (-24.6228, -29.1813) (-24.6851, -29.1604) (-24.7476, -29.1399) (-24.8103, -29.1199) (-24.8732, -29.1003) (-24.9364, -29.0812) (-24.9999, -29.0626) (-25.0636, -29.0445) (-25.1275, -29.0268) (-25.1916, -29.0095) (-25.256, -28.9927) (-25.3205, -28.9762) (-25.3852, -28.9601) (-25.4501, -28.9445) (-25.5152, -28.9292) (-25.5805, -28.9143) (-25.6459, -28.8998) (-25.7115, -28.8857) (-25.7774, -28.872) (-25.8433, -28.8586) (-25.9095, -28.8457) (-25.9758, -28.833) (-26.0422, -28.8208) (-26.1088, -28.8089) (-26.1756, -28.7973) (-26.2425, -28.7861) (-26.3096, -28.7753) (-26.3768, -28.7648) (-26.4442, -28.7547) (-26.5117, -28.7449) (-26.5793, -28.7354) (-26.6471, -28.7263) (-26.715, -28.7175) (-26.783, -28.709) (-26.8512, -28.7009) (-26.9195, -28.6931) (-26.9879, -28.6857) (-27.0564, -28.6785) (-27.1251, -28.6717) (-27.1938, -28.6652) (-27.2627, -28.6591) (-27.3317, -28.6532) (-27.4009, -28.6477) (-27.4701, -28.6424) (-27.5394, -28.6375) (-27.6089, -28.6329) (-27.6784, -28.6287) (-27.7481, -28.6247) (-27.8179, -28.621) (-27.8877, -28.6177) (-27.9577, -28.6146) (-28.0277, -28.6119) (-28.0979, -28.6094) (-28.1541, -28.6077) (-28.1963, -28.6066) (-28.2244, -28.6058) (-28.2385, -28.6055) knots 0 0 0 0 0 0 0.01428571 0.02857143 0.04285714 0.05714286 0.07142857 0.08571429 0.1 0.11428571 0.12857143 0.14285714 0.15714286 0.17142857 0.18571429 0.2 0.21428571 0.22857143 0.24285714 0.25714286 0.27142857 0.28571429 0.3 0.31428571 0.32857143 0.34285714 0.35714286 0.37142857 0.38571429 0.4 0.41428571 0.42857143 0.44285714 0.45714286 0.47142857 0.48571429 0.5 0.51428571 0.52857143 0.54285714 0.55714286 0.57142857 0.58571429 0.6 0.61428571 0.62857143 0.64285714 0.65714286 0.67142857 0.68571429 0.7 0.71428571 0.72857143 0.74285714 0.75714286 0.77142857 0.78571429 0.8 0.81428571 0.82857143 0.84285714 0.85714286 0.87142857 0.88571429 0.9 0.91428571 0.92857143 0.94285714 0.95714286 0.97142857 0.98571429 1 1 1 1 1 1
  arc A90 (-28.2385, -28.6055) -> (-28.9409, -29.822) centre (0, -45.72) ccw
  spline S45 degree 5 poles (-28.9409, -29.822) (-28.9335, -29.834) (-28.9188, -29.858) (-28.8967, -29.894) (-28.8672, -29.9418) (-28.83, -30.0013) (-28.7925, -30.0606) (-28.7549, -30.1197) (-28.7171, -30.1785) (-28.679, -30.2371) (-28.6408, -30.2954) (-28.6023, -30.3535) (-28.5636, -30.4114) (-28.5246, -30.469) (-28.4855, -30.5263) (-28.4461, -30.5834) (-28.4066, -30.6403) (-28.3668, -30.6968) (-28.3268, -30.7531) (-28.2865, -30.8092) (-28.2461, -30.865) (-28.2054, -30.9205) (-28.1645, -30.9757) (-28.1234, -31.0307) (-28.0821, -31.0854) (-28.0405, -31.1398) (-27.9987, -31.1939) (-27.9567, -31.2478) (-27.9145, -31.3013) (-27.872, -31.3546) (-27.8293, -31.4076) (-27.7864, -31.4602) (-27.7433, -31.5126) (-27.6999, -31.5646) (-27.6563, -31.6164) (-27.6124, -31.6678) (-27.5683, -31.7189) (-27.524, -31.7697) (-27.4795, -31.8202) (-27.4347, -31.8703) (-27.3897, -31.9201) (-27.3444, -31.9695) (-27.2989, -32.0186) (-27.2531, -32.0673) (-27.2071, -32.1157) (-27.1608, -32.1637) (-27.1143, -32.2113) (-27.0675, -32.2586) (-27.0205, -32.3055) (-26.9732, -32.352) (-26.9257, -32.3981) (-26.8778, -32.4438) (-26.8297, -32.489) (-26.7813, -32.5337) (-26.7326, -32.578) (-26.6836, -32.6219) (-26.6344, -32.6654) (-26.5849, -32.7084) (-26.5351, -32.751) (-26.4851, -32.7932) (-26.4347, -32.8347) (-26.3838, -32.8755) (-26.3326, -32.9156) (-26.2808, -32.9549) (-26.2288, -32.9936) (-26.1764, -33.0317) (-26.1238, -33.0695) (-26.071, -33.1069) (-26.018, -33.1438) (-25.9644, -33.1797) (-25.9099, -33.214) (-25.8654, -33.2397) (-25.8314, -33.2578) (-25.8083, -33.2692) (-25.7967, -33.2748) knots -1 -1 -1 -1 -1 -1 -0.98571429 -0.97142857 -0.95714286 -0.94285714 -0.92857143 -0.91428571 -0.9 -0.88571429 -0.87142857 -0.85714286 -0.84285714 -0.82857143 -0.81428571 -0.8 -0.78571429 -0.77142857 -0.75714286 -0.74285714 -0.72857143 -0.71428571 -0.7 -0.68571429 -0.67142857 -0.65714286 -0.64285714 -0.62857143 -0.61428571 -0.6 -0.58571429 -0.57142857 -0.55714286 -0.54285714 -0.52857143 -0.51428571 -0.5 -0.48571429 -0.47142857 -0.45714286 -0.44285714 -0.42857143 -0.41428571 -0.4 -0.38571429 -0.37142857 -0.35714286 -0.34285714 -0.32857143 -0.31428571 -0.3 -0.28571429 -0.27142857 -0.25714286 -0.24285714 -0.22857143 -0.21428571 -0.2 -0.18571429 -0.17142857 -0.15714286 -0.14285714 -0.12857143 -0.11428571 -0.1 -0.08571429 -0.07142857 -0.05714286 -0.04285714 -0.02857143 -0.01428571 0 0 0 0 0 0
  line L45 (-25.7967, -33.2748) -> (-25.7792, -33.2833)
  arc A91 (-25.1645, -34.9274) -> (-25.7792, -33.2833) centre (-26.3317, -34.4269) ccw
  arc A92 (-25.1645, -34.9274) -> (-25.4255, -35.5575) centre (0, -45.72) ccw
  arc A93 (-27.0227, -36.2854) -> (-25.4255, -35.5575) centre (-26.6048, -35.0862) ccw
  line L46 (-27.0227, -36.2854) -> (-27.0411, -36.279)
  spline S46 degree 5 poles (-27.0411, -36.279) (-27.0533, -36.2748) (-27.0777, -36.2666) (-27.1145, -36.2553) (-27.1642, -36.242) (-27.2269, -36.2277) (-27.2902, -36.2152) (-27.3538, -36.2038) (-27.4176, -36.1929) (-27.4815, -36.1825) (-27.5455, -36.1724) (-27.6097, -36.1629) (-27.674, -36.1542) (-27.7386, -36.1462) (-27.8034, -36.1392) (-27.8684, -36.1329) (-27.9336, -36.1273) (-27.9989, -36.1222) (-28.0644, -36.1177) (-28.1299, -36.1136) (-28.1956, -36.11) (-28.2613, -36.1069) (-28.3272, -36.1043) (-28.3932, -36.1022) (-28.4593, -36.1007) (-28.5255, -36.0996) (-28.5918, -36.0991) (-28.6582, -36.099) (-28.7247, -36.0994) (-28.7913, -36.1002) (-28.858, -36.1014) (-28.9247, -36.1031) (-28.9916, -36.1051) (-29.0585, -36.1077) (-29.1254, -36.1106) (-29.1925, -36.114) (-29.2596, -36.1177) (-29.3268, -36.1219) (-29.394, -36.1265) (-29.4613, -36.1315) (-29.5287, -36.1368) (-29.5961, -36.1426) (-29.6636, -36.1487) (-29.7311, -36.1552) (-29.7987, -36.1621) (-29.8664, -36.1694) (-29.9341, -36.177) (-30.0018, -36.185) (-30.0696, -36.1934) (-30.1374, -36.2021) (-30.2053, -36.2112) (-30.2732, -36.2206) (-30.3411, -36.2304) (-30.4091, -36.2406) (-30.4771, -36.2511) (-30.5451, -36.2619) (-30.6132, -36.2731) (-30.6813, -36.2846) (-30.7495, -36.2965) (-30.8176, -36.3087) (-30.8858, -36.3213) (-30.9541, -36.3341) (-31.0223, -36.3473) (-31.0906, -36.3609) (-31.1589, -36.3747) (-31.2272, -36.3889) (-31.2955, -36.4034) (-31.3639, -36.4183) (-31.4322, -36.4334) (-31.5006, -36.4489) (-31.569, -36.4647) (-31.6238, -36.4776) (-31.6648, -36.4874) (-31.6922, -36.494) (-31.7059, -36.4973) knots 0 0 0 0 0 0 0.01428571 0.02857143 0.04285714 0.05714286 0.07142857 0.08571429 0.1 0.11428571 0.12857143 0.14285714 0.15714286 0.17142857 0.18571429 0.2 0.21428571 0.22857143 0.24285714 0.25714286 0.27142857 0.28571429 0.3 0.31428571 0.32857143 0.34285714 0.35714286 0.37142857 0.38571429 0.4 0.41428571 0.42857143 0.44285714 0.45714286 0.47142857 0.48571429 0.5 0.51428571 0.52857143 0.54285714 0.55714286 0.57142857 0.58571429 0.6 0.61428571 0.62857143 0.64285714 0.65714286 0.67142857 0.68571429 0.7 0.71428571 0.72857143 0.74285714 0.75714286 0.77142857 0.78571429 0.8 0.81428571 0.82857143 0.84285714 0.85714286 0.87142857 0.88571429 0.9 0.91428571 0.92857143 0.94285714 0.95714286 0.97142857 0.98571429 1 1 1 1 1 1
  arc A94 (-31.7059, -36.4973) -> (-32.0694, -37.8541) centre (0, -45.72) ccw
  spline S47 degree 5 poles (-32.0694, -37.8541) (-32.0592, -37.8638) (-32.0388, -37.8832) (-32.0082, -37.9123) (-31.9672, -37.9508) (-31.9159, -37.9987) (-31.8644, -38.0463) (-31.8128, -38.0936) (-31.761, -38.1406) (-31.7091, -38.1873) (-31.657, -38.2338) (-31.6048, -38.2799) (-31.5524, -38.3258) (-31.4999, -38.3714) (-31.4473, -38.4166) (-31.3945, -38.4616) (-31.3416, -38.5062) (-31.2885, -38.5506) (-31.2353, -38.5946) (-31.1819, -38.6384) (-31.1284, -38.6818) (-31.0747, -38.7249) (-31.0209, -38.7677) (-30.967, -38.8101) (-30.9129, -38.8522) (-30.8587, -38.894) (-30.8043, -38.9355) (-30.7498, -38.9767) (-30.6952, -39.0174) (-30.6404, -39.0579) (-30.5854, -39.098) (-30.5303, -39.1378) (-30.4751, -39.1772) (-30.4197, -39.2162) (-30.3642, -39.2549) (-30.3085, -39.2932) (-30.2527, -39.3312) (-30.1968, -39.3688) (-30.1407, -39.406) (-30.0844, -39.4428) (-30.0281, -39.4793) (-29.9715, -39.5153) (-29.9149, -39.5509) (-29.858, -39.5862) (-29.8011, -39.621) (-29.7439, -39.6554) (-29.6867, -39.6893) (-29.6293, -39.7229) (-29.5717, -39.756) (-29.514, -39.7887) (-29.4561, -39.8209) (-29.3981, -39.8527) (-29.3399, -39.8839) (-29.2816, -39.9146) (-29.2231, -39.9447) (-29.1644, -39.9744) (-29.1056, -40.0037) (-29.0467, -40.0325) (-28.9876, -40.0608) (-28.9283, -40.0885) (-28.8689, -40.1155) (-28.8092, -40.1418) (-28.7493, -40.1672) (-28.6892, -40.1918) (-28.6289, -40.2157) (-28.5684, -40.239) (-28.5078, -40.2619) (-28.4472, -40.2844) (-28.3864, -40.3063) (-28.3253, -40.3271) (-28.2639, -40.3461) (-28.2142, -40.3594) (-28.1766, -40.368) (-28.1514, -40.3732) (-28.1388, -40.3756) knots -1 -1 -1 -1 -1 -1 -0.98571429 -0.97142857 -0.95714286 -0.94285714 -0.92857143 -0.91428571 -0.9 -0.88571429 -0.87142857 -0.85714286 -0.84285714 -0.82857143 -0.81428571 -0.8 -0.78571429 -0.77142857 -0.75714286 -0.74285714 -0.72857143 -0.71428571 -0.7 -0.68571429 -0.67142857 -0.65714286 -0.64285714 -0.62857143 -0.61428571 -0.6 -0.58571429 -0.57142857 -0.55714286 -0.54285714 -0.52857143 -0.51428571 -0.5 -0.48571429 -0.47142857 -0.45714286 -0.44285714 -0.42857143 -0.41428571 -0.4 -0.38571429 -0.37142857 -0.35714286 -0.34285714 -0.32857143 -0.31428571 -0.3 -0.28571429 -0.27142857 -0.25714286 -0.24285714 -0.22857143 -0.21428571 -0.2 -0.18571429 -0.17142857 -0.15714286 -0.14285714 -0.12857143 -0.11428571 -0.1 -0.08571429 -0.07142857 -0.05714286 -0.04285714 -0.02857143 -0.01428571 0 0 0 0 0 0
  line L47 (-28.1388, -40.3756) -> (-28.1196, -40.3792)
  arc A95 (-27.1003, -41.8082) -> (-28.1196, -40.3792) centre (-28.3573, -41.6268) ccw
  circle A96 centre (0, -45.72) radius 1.4986
sketch "Sketch4" plane through (0, 0, 10.16) normal (0, 0, 1) x (-1, 0, 0)
  circle A0 centre (0, -45.72) radius 3.81
  circle A1 centre (39.5947, 22.86) radius 1.4986
  line L0 (39.5947, 22.86) -> (39.5947, 21.209)
  line L1 (39.5947, 21.209) -> (39.5947, 22.86)
  line L2 (38.0328, 22.86) -> (39.5947, 22.86)
  circle A2 centre (39.5947, 22.86) radius 3.81
  line L3 (-41.148, 22.86) -> (-39.624, 22.86)
  line L4 (-39.624, 22.86) -> (-39.624, 20.9701)
  circle A3 centre (0, 0) radius 3.81
  point P0 (0, -45.72)
  dimension "d35" = 7.62
  dimension "d36" = 7.62
  dimension "d38" = 7.62
  constraint coincident P0 A0.centre
  constraint coincident A1.centre L0.start
  constraint vertical L0
  constraint perpendicular L1 L2
  constraint horizontal L3
  constraint perpendicular L3 L4
  constraint coincident A3.centre origin
  measures "d35" diameter of A0
  measures "d36" diameter of A2
  measures "d38" diameter of A3
extrude "Extrude3" add sketch "Sketch4" along normal blind 5.08 contours A2 | A3 bodies 3 makes body 6
extrude "Extrude3'" add sketch "Sketch4" along normal blind 5.08 contours A0 sketch seen with x (1, 0, 0) y (0, 1, 0) z (0, 0, 1) at (0, -45.72, 0) bodies 5 in component "Spur Gear (24 teeth)"
sketch "Sketch5" plane through (0, 0, 15.24) normal (0, 0, 1) x (-1, 0, 0)
  circle A0 centre (39.5947, 22.86) radius 3.81
  circle A1 centre (0, 0) radius 3.81 construction
  circle A2 centre (39.5947, 22.86) radius 3.81 construction
  circle A3 centre (-39.6234, 22.8516) radius 3.81
  circle A4 centre (0, -45.72) radius 3.81
  line L0 (41.4997, 19.5604) -> (11.43, 2.1997)
  line L1 (37.6897, 26.1596) -> (7.5501, 8.7584)
  line L2 (-7.7083, 8.7691) -> (-37.7138, 26.1485)
  line L3 (-41.5269, 19.5511) -> (-11.4363, 2.1973)
  line L4 (3.81, -10.9985) -> (3.81, -45.72)
  line L5 (-3.81, -45.72) -> (-3.81, -11.0045)
  arc A5 (11.43, 2.1997) -> (3.81, -10.9985) centre (19.05, -10.9985) ccw
  arc A6 (-3.81, -11.0045) -> (-11.4363, 2.1973) centre (-19.05, -11.0045) ccw
  arc A7 (-7.7083, 8.7691) -> (7.5501, 8.7584) centre (-0.0699, 21.9567) ccw
  dimension "d44" = 7.62
  dimension "d45" = 7.62
  dimension "d46" = 7.62
  dimension "d47" = 7.62
  dimension "d48" = 15.24
  dimension "d49" = 15.24
  dimension "d50" = 15.24
  constraint coincident A1.centre origin
  constraint concentric A0 A2
  constraint coincident A2 L0.start
  constraint coincident A2 L1.start
  constraint tangent A1 L1
  constraint tangent A1 L0
  constraint tangent A2 L1
  constraint tangent A2 L0
  constraint coincident A3 L2.end
  constraint coincident A3 L3.start
  constraint tangent A1 L3
  constraint tangent A3 L3
  constraint tangent A3 L2
  constraint coincident A4 L4.end
  constraint vertical L4
  constraint coincident A4 L5.start
  constraint tangent A1 L5
  constraint tangent A4 L5
  constraint tangent A4 L4
  constraint tangent L0 A5
  constraint tangent L4 A5
  constraint tangent L5 A6
  constraint tangent L3 A6
  constraint tangent L1 A7
  constraint tangent L2 A7
  measures "d44" diameter of A1
  measures "d45" diameter of A2
  measures "d46" diameter of A3
  measures "d47" diameter of A4
  measures "d48" radius of A5
  measures "d49" radius of A6
  measures "d50" radius of A7
extrude "Extrude4" add sketch "Sketch5" along normal blind 5.08 bodies 3 6
sketch "Sketch6" plane through (0, 0, 20.32) normal (0, 0, 1) x (-1, 0, 0)
  arc A0 (-37.7138, 26.1485) -> (-41.5269, 19.5511) centre (-39.6234, 22.8516) ccw
  line L0 (-41.5269, 19.5511) -> (-11.4363, 2.1973)
  arc A1 (-3.81, -11.0045) -> (-11.4363, 2.1973) centre (-19.05, -11.0045) ccw
  line L1 (-3.81, -11.0045) -> (-3.81, -45.72)
  arc A2 (-3.81, -45.72) -> (3.81, -45.72) centre (0, -45.72) ccw
  line L2 (3.81, -45.72) -> (3.81, -10.9985)
  arc A3 (11.43, 2.1997) -> (3.81, -10.9985) centre (19.05, -10.9985) ccw
  line L3 (11.43, 2.1997) -> (41.4997, 19.5604)
  arc A4 (41.4997, 19.5604) -> (37.6897, 26.1596) centre (39.5947, 22.86) ccw
  line L4 (37.6897, 26.1596) -> (7.5501, 8.7584)
  arc A5 (-7.7083, 8.7691) -> (7.5501, 8.7584) centre (-0.0699, 21.9567) ccw
  line L5 (-7.7083, 8.7691) -> (-37.7138, 26.1485)
  circle A6 centre (0, 0) radius 6.35
  dimension "d55" = 12.7
  constraint coincident A6.centre origin
  measures "d55" diameter of A6
extrude "Extrude5" add sketch "Sketch6" along normal blind 40.64 contours A6 bodies 3
move_body "Move1" bodies 3 to x (1, 0, 0) y (0, 1, 0) z (0, 0, 1) at (0, 109.22, 0)
sketch "Sketch7" plane through (0, 0, 15.24) normal (0, 0, 1) x (-1, 0, 0)
  circle A0 centre (39.5947, 22.86) radius 3.81
  circle A1 centre (39.5947, 22.86) radius 3.81
  circle A2 centre (0, 0) radius 3.81
  circle A3 centre (0, -45.72) radius 3.81
  dimension "d58" = 7.62
  dimension "d59" = 7.62
  dimension "d60" = 7.62
  constraint concentric A0 A1
  constraint coincident A2.centre origin
  measures "d58" diameter of A1
  measures "d59" diameter of A2
  measures "d60" diameter of A3
extrude "Extrude3''" cut sketch "Sketch7" against normal blind 7.62 sketch seen with x (0.965926, -0.258819, 0) y (0.258819, 0.965926, 0) z (0, 0, 1) at (0, 0, 0) bodies 4 in component "Spur Gear (12 teeth)"
extrude "Extrude4'" cut sketch "Sketch7" against normal blind 7.62 sketch seen with x (-0.5, -0.866025, 0) y (0.866025, -0.5, 0) z (0, 0, 1) at (0, -45.72, 0) bodies 5 in component "Spur Gear (24 teeth)"
component "Spur Gear (60 teeth)" placed x (1, 0, 0) y (0, 1, 0) z (0, 0, 1) at (0, 0, 0)
component "Spur Gear (12 teeth)" placed x (0.965926, 0.258819, 0) y (-0.258819, 0.965926, 0) z (0, 0, 1) at (0, 0, 0)
component "Spur Gear (24 teeth)" placed x (-0.5, 0.866025, 0) y (-0.866025, -0.5, 0) z (0, 0, 1) at (-39.5947, -22.86, 0)
component "Spur Gear (24 teeth)" placed x (1, 0, 0) y (0, 1, 0) z (0, 0, 1) at (0, 45.72, 0)
component "Spur Gear (24 teeth)" placed x (-0.5, -0.866025, 0) y (0.866025, -0.5, 0) z (0, 0, 1) at (39.5947, -22.86, 0)
equation "gearThickness = 0.4 in"
equation "holeDia = 0.118 in"
equation "d13 = gearThickness"
equation "carrierHoleDia = 0.3 in"
equation "outputShaft = 0.5 in"
equation "d35 = carrierHoleDia"
equation "d36 = carrierHoleDia"
equation "d38 = carrierHoleDia"
equation "carrierStrutHeight = 0.2 in"
equation "d40 = carrierStrutHeight"
equation "d42 = carrierStrutHeight"
equation "d44 = carrierHoleDia"
equation "d45 = carrierHoleDia"
equation "d46 = carrierHoleDia"
equation "d47 = carrierHoleDia"
equation "carrierMainHeight = 0.2 in"
equation "outputShaftHeight = 1.6 in"
equation "d53 = carrierMainHeight"
equation "d55 = outputShaft"
equation "d56 = outputShaftHeight"
equation "d58 = carrierHoleDia"
equation "d59 = carrierHoleDia"
equation "d60 = carrierHoleDia"
